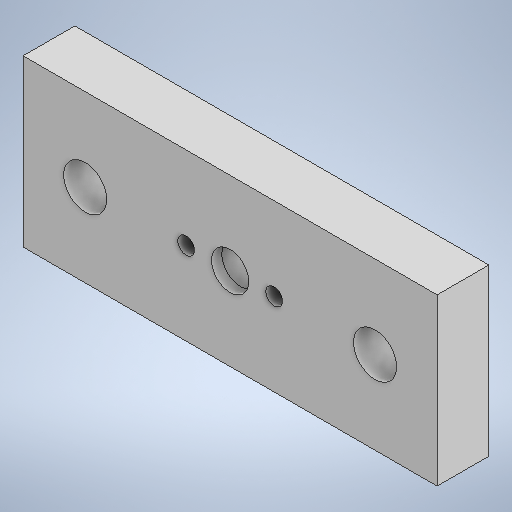
# Autodesk Inventor part: 13042026-09
Saved by Autodesk Inventor 2025.2 (Build 292293000, 293)
## iProperties
Created: 2026-05-06
Part Number: 13042026-09
Material: Generic
Document SubType Name: Modeling
Designer: Oski
Density: 1 g/cm^3
Appearance: Default
Author: Oski
Autodesk Inventor part; units mm, degrees
ref_plane "YZ Plane" through (0, 0, 0) normal (1, 0, 0) x (0, 1, 0)
ref_plane "XZ Plane" through (0, 0, 0) normal (0, 1, 0) x (-1, 0, 0)
ref_plane "XY Plane" through (0, 0, 0) normal (0, 0, 1) x (1, 0, 0)
sketch "Sketch1" plane through (0, 0, 0) normal (0, 0, 1) x (1, 0, 0)
  line L0 (-40, 16) -> (40, 16)
  line L1 (40, 16) -> (40, -16)
  line L2 (40, -16) -> (-40, -16)
  line L3 (-40, -16) -> (-40, 16)
  line L4 (-40, 16) -> (40, -16) construction
  line L5 (40, 16) -> (-40, -16) construction
  point P0 (0, 0)
  dimension "d0" = 80
  dimension "d1" = 32
  constraints: 12 end point, 2 midpoint, 2 parallel, 1 horizontal, 1 perpendicular
  measures "d0" distance of L0.start L0.end
  measures "d1" distance of L0.end L1.end
extrude "Extrusion1" add sketch "Sketch1" along normal blind 10
sketch "Sketch2" plane through (0, 0, 10) normal (0, 0, 1) x (1, 0, 0)
  line L0 (-28, 0) -> (-40, 0)
  line L1 (-40, 16) -> (-40, -16) projected
  line L2 (28, 0) -> (40, 0)
  line L3 (40, -16) -> (40, 16) projected
  point P0 (0, 0)
  dimension "d4" = 56
  constraints: 4 end point, 2 horizontal, 2 midpoint, 1 collinear, 1 point on line
  measures "d4" distance of L2.start L0.start
hole "Hole1" at (28, 0, 10) at (-28, 0, 10) direction (0, 0, -1) diameter 8.3 end through all
sketch "Sketch4" plane through (0, 0, 0) normal (0, 0, -1) x (-1, 0, 0)
  line L0 (-8.5, 0) -> (-40, 0) construction
  line L1 (8.5, 0) -> (40, 0) construction
  line L2 (40, 16) -> (40, -16) projected
  line L3 (-40, -16) -> (-40, 16) projected
  line L4 (-40, 0) -> (40, 0)
  point P0 (0, 0)
  dimension "d13" = 8.5
  constraints: 6 end point, 4 midpoint, 2 horizontal, 2 point on line, 1 collinear
  measures "d13" distance of L0.start point (0, 0)
hole "Hole2" at (-8.5, 0, 0) at (8.5, 0, 0) direction (0, 0, 1) diameter 3.2 end through all counterbore diameter 6.2 counterbore depth 2.2
sketch "Sketch5" plane through (0, 0, 0) normal (0, 0, -1) x (-1, 0, 0)
  point P0 (0, 0)
  point P1 (0, 0)
  constraints: 1 coincident
hole "Hole3" at (0, 0, 0) direction (0, 0, 1) diameter 7.2 end through all counterbore diameter 8 counterbore depth 8
body "Solid1"
